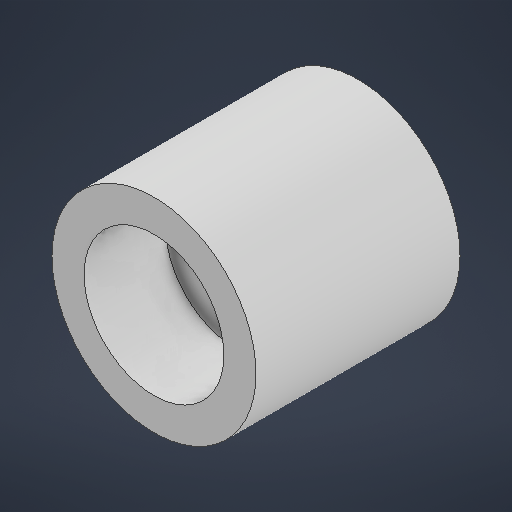
# Autodesk Inventor part: Shaft Coupler
Saved by Autodesk Inventor 2025.3 (Build 293356030, 356C)
## iProperties
Created: 2025-10-14
Part Number: Shaft Coupler
Material: Generic
Document SubType Name: Modeling
Designer: yo
Density: 1 g/cm^3
Appearance: Default
Author: yo
Autodesk Inventor part; units mm, degrees
ref_plane "YZ Plane" through (0, 0, 0) normal (1, 0, 0) x (0, 1, 0)
ref_plane "XZ Plane" through (0, 0, 0) normal (0, 1, 0) x (-1, 0, 0)
ref_plane "XY Plane" through (0, 0, 0) normal (0, 0, 1) x (1, 0, 0)
sketch "Sketch1" plane through (0, 0, 0) normal (0, 0, 1) x (1, 0, 0)
  circle A0 centre (0, 0) radius 3.425
  circle A1 centre (0, 0) radius 5
  dimension "d0" = 6.85
  dimension "d1" = 10
  constraints: 2 centre point, 2 coincident
  measures "d0" diameter of A0
  measures "d1" diameter of A1
extrude "Extrusion1" add sketch "Sketch1" along normal blind 4
extrude "Extrusion2" add sketch "Sketch1" against normal blind 6 contours A0 | A1
sketch "Sketch2" plane through (0, 0, -6) normal (0, 0, -1) x (-1, 0, 0)
  circle A0 centre (0, 0) radius 2.5
  line L0 (-1.5, 2) -> (1.5, 2)
  dimension "d6" = 5
  dimension "d7" = 0.5
  constraints: 2 end point, 2 point on circle, 1 centre point, 1 coincident, 1 horizontal
  measures "d6" diameter of A0
  measures "d7" distance edge to line of A0 L0
extrude "Extrusion3" cut sketch "Sketch2" against normal blind 4 contours A0 L0 picked at (0.1119, 0.5076)
body "Solid1"
